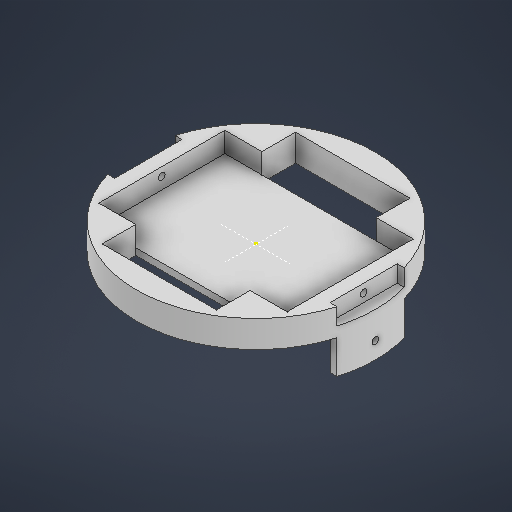
# Autodesk Inventor part: 003-001
Saved by Autodesk Inventor 2026 (Build 300175000, 175)
## iProperties
Created: 2026-04-19
Part Number: 003-001
Material: Ogólny
Document SubType Name: Modeling
Designer: Patryk Lombardo
Density: 1 g/cm^3
Appearance: Domyślna
Author: Patryk Lombardo
Autodesk Inventor part; units mm, degrees
ref_plane "YZ Plane" through (0, 0, 0) normal (1, 0, 0) x (0, 1, 0)
ref_plane "XZ Plane" through (0, 0, 0) normal (0, 1, 0) x (-1, 0, 0)
ref_plane "XY Plane" through (0, 0, 0) normal (0, 0, 1) x (1, 0, 0)
sketch "Szkic1" plane through (0, 0, 0) normal (0, 1, 0) x (-1, 0, 0)
  circle A0 centre (0, 0) radius 35.5
  line L0 (0, 18.75) -> (0, -18.75) construction
  line L1 (-28, 0) -> (28, 0) construction
  line L2 (-28, -18.75) -> (28, -18.75)
  line L3 (-28, 18.75) -> (-28, -18.75)
  line L4 (28, 18.75) -> (28, -18.75)
  line L5 (0, 18.75) -> (28, 18.75)
  line L6 (0, 18.75) -> (-28, 18.75)
  line L7 (0, 18.75) -> (0, 28.75) construction
  line L8 (17, 28.75) -> (-17, 28.75)
  line L9 (17, 28.75) -> (17, 18.75)
  line L10 (-17, 28.75) -> (-17, 18.75)
  line L11 (0, -18.75) -> (0, -28.75) construction
  line L12 (-17, -28.75) -> (17, -28.75)
  line L13 (17, -28.75) -> (17, -18.75)
  line L14 (-17, -28.75) -> (-17, -18.75)
  dimension "d0" = 71
  dimension "d1" = 37.5
  dimension "d2" = 56
  dimension "d3" = 10
  dimension "d4" = 34
  dimension "d5" = 10
  dimension "d6" = 34
  constraints: 30 end point, 7 midpoint, 5 horizontal, 5 vertical, 4 point on line, 3 perpendicular, 2 coincident, 1 centre point, 1 collinear
  measures "d0" diameter of A0
  measures "d1" distance of L0.start L0.end
  measures "d2" distance of L1.start L1.end
  measures "d3" distance of L0.start L7.end
  measures "d4" distance of L8.start L8.end
  measures "d5" distance of L0.end L11.end
  measures "d6" distance of L12.start L12.end
extrude "Wyciągnięcie proste1" add sketch "Szkic1" along normal blind 2 contours L3 L6 L5 L4 L2
extrude "Wyciągnięcie proste2" add sketch "Szkic1" along normal blind 8
sketch "Szkic2" plane through (0, 0, 0) normal (0, -1, 0) x (1, 0, 0)
  line L0 (32, 0) -> (-32, 0) construction
  circle A0 centre (0, 0) radius 35.5
  line L1 (-32, -10) -> (-32, 10)
  line L2 (32, -10) -> (32, 10)
  line L3 (32, -10) -> (34.0624, -10)
  line L4 (32, 10) -> (34.0624, 10)
  line L5 (-32, -10) -> (-34.0624, -10)
  line L6 (-32, 10) -> (-34.0624, 10)
  dimension "d11" = 64
  dimension "d12" = 71
  dimension "d13" = 20
  dimension "d14" = 20
  constraints: 14 end point, 4 horizontal, 4 point on circle, 3 midpoint, 2 coincident, 2 vertical, 1 centre point, 1 parallel
  measures "d11" distance of L0.start L0.end
  measures "d12" diameter of A0
  measures "d13" distance of L1.start L1.end
  measures "d14" distance of L2.start L2.end
extrude "Wyciągnięcie proste3" add sketch "Szkic2" along normal blind 10 contours A0 L3 L2 L4 | L6 L1 L5 A0
sketch "Szkic3" plane through (32, 0, -10) normal (-1, 0, 0) x (0, 0, 1)
  line L0 (10, 0) -> (10, -5) construction
  circle A0 centre (10, -5) radius 1
  dimension "d17" = 5
  dimension "d18" = 2
  constraints: 2 end point, 1 centre point, 1 coincident, 1 vertical
  measures "d17" distance of L0.start L0.end
  measures "d18" diameter of A0
extrude "Wyciągnięcie proste4" cut sketch "Szkic3" along normal through all both and the other way through all
sketch "Szkic4" plane through (0, 2, 0) normal (0, 1, 0) x (1, 0, 0)
  line L0 (-10.2735, 0) -> (10.2735, 0) construction
  line L1 (0, 9.2596) -> (0, -9.2596) construction
  point P0 (0, 0)
  constraints: 4 end point, 2 midpoint, 1 horizontal, 1 vertical
sketch "Szkic5" plane through (0, 8, 0) normal (0, 1, 0) x (1, 0, 0)
  line L0 (32, 0) -> (-32, 0) construction
  circle A0 centre (0, 0) radius 35.5
  line L1 (-32, -10) -> (-32, 10)
  line L2 (32, -10) -> (32, 10)
  line L3 (32, -10) -> (34.0624, -10)
  line L4 (32, 10) -> (34.0624, 10)
  line L5 (-32, -10) -> (-34.0624, -10)
  line L6 (-32, 10) -> (-34.0624, 10)
  dimension "d21" = 64
  dimension "d22" = 71
  dimension "d23" = 20
  dimension "d24" = 20
  constraints: 14 end point, 4 horizontal, 4 point on circle, 3 coincident, 3 midpoint, 2 vertical, 1 centre point, 1 parallel
  measures "d21" distance of L0.start L0.end
  measures "d22" diameter of A0
  measures "d23" distance of L1.start L1.end
  measures "d24" distance of L2.start L2.end
extrude "Wyciągnięcie proste5" cut sketch "Szkic5" against normal blind 5 contours A0 L3 L2 L4 | L6 L1 L5 A0
sketch "Szkic6" plane through (32, 8, 10) normal (1, 0, 0) x (0, 0, -1)
  line L0 (10, -8) -> (10, -2.5) construction
  circle A0 centre (10, -2.5) radius 1
  dimension "d27" = 5.5
  dimension "d28" = 2
  constraints: 2 end point, 1 centre point, 1 coincident, 1 vertical
  measures "d27" distance of L0.start L0.end
  measures "d28" diameter of A0
extrude "Wyciągnięcie proste6" cut sketch "Szkic6" against normal through all
